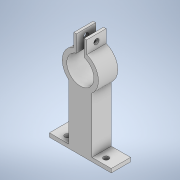
# Autodesk Inventor part: base_motor
Saved by Autodesk Inventor 2022 (Build 260153000, 153)
## iProperties
Created: 2022-03-03
Part Number: base_motor
Material: Generic
Document SubType Name: Modeling
Designer: katha
Density: 1 g/cm^3
Appearance: Default
Author: katha
Autodesk Inventor part; units mm, degrees
ref_plane "YZ Plane" through (0, 0, 0) normal (1, 0, 0) x (0, 1, 0)
ref_plane "Work Plane3" through (158.3589, -41.348, 102.8428) normal (0, 0, -1) x (-1, 0, 0)
sketch "Sketch3" plane through (158.3589, -41.348, 102.8428) normal (0, 0, -1) x (-1, 0, 0)
  circle A0 centre (0, 0) radius 10.5 projected
  arc A1 (-3, 10.0623) -> (3, 10.0623) centre (0, 0) ccw
  line L0 (0, 0) -> (0, 16.5106) construction
  line L1 (5, 13.0767) -> (5, 23.0767)
  line L2 (3, 10.0623) -> (3, 23.0767)
  line L3 (5, 23.0767) -> (3, 23.0767)
  line L4 (-5, 13.0767) -> (-5, 23.0767)
  line L5 (-3, 10.0623) -> (-3, 23.0767)
  line L6 (-5, 23.0767) -> (-3, 23.0767)
  arc A2 (-5, 13.0767) -> (5, 13.0767) centre (0, 0) ccw
  point P0 (158.3589, 41.348)
  dimension "d8" = 0
  dimension "d30" = 10
  dimension "d31" = 2
  dimension "d32" = 3
  dimension "d33" = 14
  constraints: 14 end point, 4 point on circle, 4 symmetric about line, 2 centre point, 2 vertical, 1 horizontal, 1 parallel
  measures "d8" radial gap between concentric circles of A0 A1
  measures "d30" distance of L1.start L1.end
  measures "d31" distance between parallel lines of L1 L2
  measures "d32" distance between parallel lines of L2 L0
  measures "d33" radius of A2
extrude "Extrusion2" add sketch "Sketch3" against normal blind 15 contours A0 L2 L3 L1 A2 L4 L6 L5
sketch "Sketch5" plane through (158.3589, -41.348, 102.8428) normal (0, 0, -1) x (-1, 0, 0)
  line L0 (-41.6411, -56.9287) -> (358.3589, -56.9287) projected
  arc A0 (-2.5, 13.775) -> (2.5, 13.775) centre (0, 0) ccw projected
  line L1 (0, -14) -> (0, -56.9287) construction
  line L2 (9, -10.7238) -> (9, -56.9287)
  line L3 (-9, -10.7238) -> (-9, -56.9287)
  point P0 (158.3589, 41.348)
  point P1 (-9, -10.7238)
  point P2 (-9, -56.9287)
  dimension "d19" = 9
  constraints: 6 end point, 2 perpendicular, 2 point on circle, 2 point on line, 2 symmetric about line
  measures "d19" distance between parallel lines of L2 L1
extrude "Extrusion4" add sketch "Sketch5" against normal blind 15
ref_plane "Work Plane5" through (0, -98.2767, 225.7428) normal (0, 1, 0) x (-1, 0, 0)
sketch "Sketch7" plane through (0, -98.2767, 225.7428) normal (0, 1, 0) x (-1, 0, 0)
  circle A0 centre (-143.3589, -112.9) radius 2 projected
  circle A1 centre (-173.3589, -112.9) radius 2 projected
  line L0 (-134.3589, -107.9) -> (-182.3589, -107.9)
  line L1 (-182.3589, -107.9) -> (-182.3589, -122.9)
  line L2 (-182.3589, -122.9) -> (-134.3589, -122.9)
  line L3 (-134.3589, -122.9) -> (-134.3589, -107.9)
  line L4 (-144.3589, -107.9) -> (-155.8589, -107.9) projected
  point P0 (0, -225.7428)
  point P1 (-149.3589, -107.9)
  dimension "d23" = 48
  dimension "d24" = 15
  dimension "d25" = 9
  constraints: 8 end point, 2 parallel, 1 collinear, 1 horizontal, 1 perpendicular
  measures "d23" distance of L2.end L1.end
  measures "d24" distance of L2.end L0.start
  measures "d25" distance from line of L3 A0.centre
extrude "Extrusion5" add sketch "Sketch7" along normal blind 3
sketch "Sketch8" plane through (153.3589, -28.2713, 102.8428) normal (-1, 0, 0) x (0, 0, 1)
  line L0 (0, 0) -> (0, 10) projected
  line L1 (0, 10) -> (15, 10) projected
  line L2 (0, 5) -> (15, 5) construction
  line L3 (0, 10) -> (15, 10) projected
  line L4 (7.5, 10) -> (7.5, 0) construction
  circle A0 centre (7.5, 5) radius 2
  point P0 (-102.8428, 28.2713)
  dimension "d34" = 4
  constraints: 4 end point, 3 midpoint, 1 centre point, 1 horizontal, 1 vertical
  measures "d34" diameter of A0
extrude "Extrusion6" cut sketch "Sketch8" against normal blind 10
body "Solid2"
